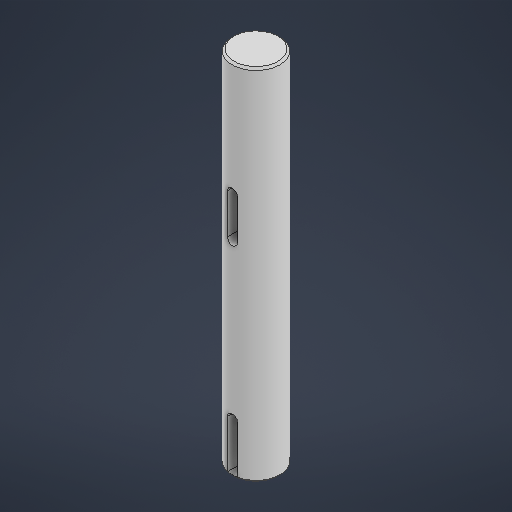
# Autodesk Inventor part: eixo 5
Saved by Autodesk Inventor 2026.2 (Build 302298000, 298)
## iProperties
Created: 2026-09-11
Part Number: eixo 5
Material: Genérico
Document SubType Name: Modeling
Designer: IFSP
Density: 1 g/cm^3
Appearance: Padrão
Author: IFSP
Autodesk Inventor part; units mm, degrees
ref_plane "YZ Plane" through (0, 0, 0) normal (1, 0, 0) x (0, 1, 0)
sketch "Esboço1" plane through (0, 0, 0) normal (0, 1, 0) x (-1, 0, 0)
  circle A0 centre (0, 0) radius 6
  dimension "d0" = 12
  constraints: 1 centre point, 1 coincident
  measures "d0" diameter of A0
extrude "Extrusão1" add sketch "Esboço1" along normal blind 90
chamfer "Chanfro1" distance 0.5 angle 45 1 edges at (6, 90, 0) measured on face at (0.7092, 90, 1.4219)
chamfer "Chanfro2" distance 0.5 angle 45 1 edges at (6, 0, 0) measured on face at (0.7092, 0, 1.4219)
ref_plane "Plano de trabalho1" through (0, 0, -6) normal (0, 0, 1) x (1, 0, 0)
ref_plane "Plano de trabalho2" through (0, 0, 6) normal (0, 0, 1) x (1, 0, 0)
sketch "Esboço2" plane through (0, 0, 6) normal (0, 0, 1) x (1, 0, 0)
  line L0 (6, 89.5) -> (-6, 89.5) construction
  line L1 (6, 89.5) -> (6, 61.5) construction
  line L2 (6, 0.5) -> (6, 89.5) construction
  line L3 (6, 61.5) -> (6, 51.5) construction
  line L4 (6, 0.5) -> (6, 12.5) construction
  line L5 (0, 61.5) -> (0, 51.5) construction
  line L6 (-1.25, 61.5) -> (-1.25, 51.5)
  line L7 (1.25, 51.5) -> (1.25, 61.5)
  arc A0 (1.25, 61.5) -> (-1.25, 61.5) centre (0, 61.5) ccw
  arc A1 (-1.25, 51.5) -> (1.25, 51.5) centre (0, 51.5) ccw
  line L8 (0, 12.5) -> (0, 0.5) construction
  line L9 (-6, 0.5) -> (6, 0.5) projected
  line L10 (-1.25, 12.5) -> (-1.25, 0.5)
  line L11 (1.25, 0.5) -> (1.25, 12.5)
  arc A2 (1.25, 12.5) -> (-1.25, 12.5) centre (0, 12.5) ccw
  arc A3 (-1.25, 0.5) -> (1.25, 0.5) centre (0, 0.5) ccw
  point P0 (0, 0)
  point P1 (0, 56.5)
  point P2 (0, 6.5)
  dimension "d9" = 28
  dimension "d10" = 10
  dimension "d11" = 12
  dimension "d12" = 2.5
  dimension "d13" = 2.5
  constraints: 22 end point, 8 point on circle, 8 tangent, 4 centre point, 3 midpoint, 3 point on line, 2 parallel, 1 vertical
  measures "d9" distance of L0.start L1.end
  measures "d10" distance of L1.end L3.end
  measures "d11" distance of L2.start L4.end
  measures "d12" diameter of A1
  measures "d13" diameter of A3
extrude "Extrusão2" cut sketch "Esboço2" against normal blind 2.5 contours A0 L7 A1 L6 | L10 A2 L11 L9
